nut+bolt v1 (Autodesk Fusion 360 design; units mm, degrees)
Autodesk Fusion 360 part; units mm, degrees
sketch "Sketch1" plane through (0, 0, 0) normal (0, 0, 1) x (1, 0, 0)
  line L0 (34.6373, 0.5077) -> (16.879, 30.2506)
  line L1 (16.879, 30.2506) -> (-17.7583, 29.7429)
  line L2 (-17.7583, 29.7429) -> (-34.6373, -0.5077)
  line L3 (-34.6373, -0.5077) -> (-16.879, -30.2506)
  line L4 (-16.879, -30.2506) -> (17.7583, -29.7429)
  line L5 (17.7583, -29.7429) -> (34.6373, 0.5077)
  dimension "d1" = 30
  measures "d1" distance of origin L5
extrude "Extrude1" add sketch "Sketch1" along normal blind 10 makes body 1
sketch "Sketch2" plane through (0, 0, 10) normal (0, 0, 1) x (-1, 0, 0)
  line L0 (-17.7583, 29.7429) -> (-34.6373, -0.5077)
  line L1 (-34.6373, -0.5077) -> (-16.879, -30.2506)
  line L2 (-16.879, -30.2506) -> (17.7583, -29.7429)
  line L3 (17.7583, -29.7429) -> (34.6373, 0.5077)
  line L4 (34.6373, 0.5077) -> (16.879, 30.2506)
  line L5 (16.879, 30.2506) -> (-17.7583, 29.7429)
  circle A0 centre (0, 0) radius 10
  dimension "d4" = 20
  constraint coincident A0.centre origin
  measures "d4" diameter of A0
extrude "Extrude2" cut sketch "Sketch2" against normal up to surface (10 mm away) contours A0 bodies 1
thread "Thread1" "ISO Metric profile 20.0 M20x2.5 6H" major diameter 20.2925 minor diameter 17.519 pitch 2.5 angle 60 modelled right hand crest width 0.6905 on face at (-9.9876, 0.4985, 3.3333) crest through (-8.7595, 0, 9.375) on bodies 1
copy_body "Body->Comp1" bodies 1 removing the originals makes body 2 in component "nut"
sketch "Sketch1 (2)" plane through (0, 0, 0) normal (0, 0, 1) x (1, 0, 0) in component "bolt"
  circle A0 centre (0, 0) radius 15
  dimension "d7" = 30
  constraint coincident A0.centre origin
  measures "d7" diameter of A0
extrude "Extrude1'" add sketch "Sketch1 (2)" along normal blind 70 separate body makes body 3 in component "bolt"
sketch "Sketch2 (2)" plane through (0, 0, 70) normal (0, 0, 1) x (-1, 0, 0) in component "bolt"
  circle A0 centre (0, 0) radius 15
  line L0 (-33.101, -32.2127) -> (11.3465, -44.7727)
  line L1 (11.3465, -44.7727) -> (44.4475, -12.56)
  line L2 (44.4475, -12.56) -> (33.101, 32.2127)
  line L3 (33.101, 32.2127) -> (-11.3465, 44.7727)
  line L4 (-11.3465, 44.7727) -> (-44.4475, 12.56)
  line L5 (-44.4475, 12.56) -> (-33.101, -32.2127)
  dimension "d10" = 40
  constraint coincident A0.centre origin
  measures "d10" distance of A0.centre L5
sketch "Sketch3" plane through (0, 0, 70) normal (0, 0, 1) x (-1, 0, 0) in component "bolt"
  circle A0 centre (0, 0) radius 15
  line L0 (-34.6024, -30.5942) -> (9.1942, -45.2637)
  line L1 (9.1942, -45.2637) -> (43.7966, -14.6694)
  line L2 (43.7966, -14.6694) -> (34.6024, 30.5942)
  line L3 (34.6024, 30.5942) -> (-9.1942, 45.2637)
  line L4 (-9.1942, 45.2637) -> (-43.7966, 14.6694)
  line L5 (-43.7966, 14.6694) -> (-34.6024, -30.5942)
  dimension "d13" = 40
  constraint coincident A0.centre origin
  measures "d13" distance of A0.centre L5
extrude "Extrude3" add sketch "Sketch3" along normal blind 20 contours A0 | L0 L1 L2 L3 L4 L5 bodies 3 in component "bolt"
thread "Thread1'" "ISO Metric profile 30.0 M30x3.5 6g" major diameter 29.7345 minor diameter 25.732 pitch 3.5 angle 60 modelled right hand crest width 0.4992 on face at (14.9255, -1.4935, 46.6667) from (0, 0, 0) to (0, 0, 30) crest through (14.8673, 0, -0.875) on bodies 3 in component "bolt"
extrude "Extrude2'" [suppressed] in component "bolt"
component "nut" placed x (1, 0, 0) y (0, 1, 0) z (0, 0, 1) at (0, 0, 0)
component "bolt" placed x (1, 0, 0) y (0, 1, 0) z (0, 0, 1) at (0, 0, 0)
named bodies: "nut"
